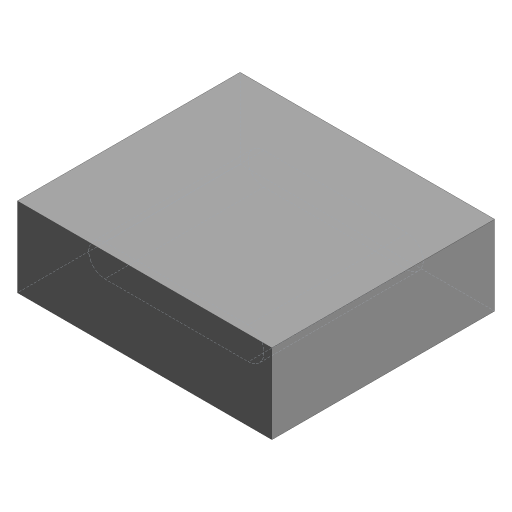
# Autodesk Inventor part: Single_Mode_Rect
Saved by Autodesk Inventor 2023 (Build 270158000, 158)
## iProperties
Part Number: Single_Mode_Rect
Material: Generic
Document SubType Name: Modeling
Designer: cssri
Appearance: Default
Author: cssri
Autodesk Inventor part; units mm, degrees
ref_plane "YZ Plane" through (0, 0, 0) normal (1, 0, 0) x (0, 1, 0)
ref_plane "XZ Plane" through (0, 0, 0) normal (0, 1, 0) x (-1, 0, 0)
ref_plane "XY Plane" through (0, 0, 0) normal (0, 0, 1) x (1, 0, 0)
sketch "Sketch1" plane through (0, 0, -15.875) normal (0, 0, 1) x (1, 0, 0)
  line L0 (-14.3205, -3.175) -> (14.3205, -3.175)
  arc A0 (14.3205, -3.175) -> (14.3205, 3.175) centre (14.3205, 0) ccw
  line L1 (14.3205, 3.175) -> (-14.3205, 3.175)
  arc A1 (-14.3205, 3.175) -> (-14.3205, -3.175) centre (-14.3205, 0) ccw
  line L2 (-14.3205, -3.175) -> (-14.3205, -3.175)
  constraints: 6 end point, 4 point on circle, 2 centre point
sketch "Sketch2" plane through (0, 0, -22.225) normal (0, 0, 1) x (1, 0, 0)
  line L0 (-25.4, -7.9375) -> (25.4, -7.9375)
  line L1 (25.4, -7.9375) -> (25.4, 7.9375)
  line L2 (25.4, 7.9375) -> (-25.4, 7.9375)
  line L3 (-25.4, 7.9375) -> (-25.4, -7.9375)
  line L4 (-25.4, -7.9375) -> (25.4, 7.9375) construction
  line L5 (25.4, -7.9375) -> (-25.4, 7.9375) construction
  point P0 (0, 0)
  constraints: 12 end point, 2 midpoint, 2 parallel, 1 horizontal, 1 perpendicular
extrude "Extrusion1" add sketch "Sketch2" along normal blind 44.45
extrude "Extrusion2" cut sketch "Sketch1" along normal blind 31.75
body "Solid1"
